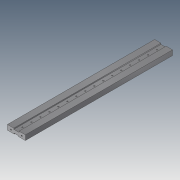
# Autodesk Inventor part: Zcolumn
Saved by Autodesk Inventor 2019 (Build 230136000, 136)
## iProperties
Created: 2018-10-03
Part Number: Zcolumn
Material: Aluminum 6061-AHC
Document SubType Name: Modeling
Designer: LillaHunden
Density: 2.7 g/cm^3
Appearance: Aluminum - Dark
Mass: 595.165 g
Surface Area: 512.389 cm^2
Volume: 220.432 cm^3
Author: LillaHunden
Autodesk Inventor part; units mm, degrees
ref_plane "YZ Plane" through (0, 0, 0) normal (1, 0, 0) x (0, 1, 0)
ref_plane "XZ Plane" through (0, 0, 0) normal (0, 1, 0) x (-1, 0, 0)
ref_plane "XY Plane" through (0, 0, 0) normal (0, 0, 1) x (1, 0, 0)
sketch "Sketch1" plane through (0, 0, 0) normal (0, 0, 1) x (1, 0, 0)
  line L0 (-83.9793, 29.5203) -> (-133.9793, 29.5203)
  line L1 (-133.9793, 29.5203) -> (-133.9793, 43.2703)
  line L2 (-133.9793, 43.2703) -> (-83.9793, 43.2703)
  line L3 (-83.9793, 43.2703) -> (-83.9793, 29.5203)
  point P0 (0, 0)
  dimension "d0" = 50
  dimension "d1" = 13.75
  constraints: 8 end point, 2 parallel, 1 horizontal, 1 perpendicular
  measures "d0" distance of L1.end L2.end
  measures "d1" distance of L0.end L1.end
extrude "Extrusion1" add sketch "Sketch1" along normal blind 410
sketch "Sketch2" plane through (-133.9793, 43.2703, 0) normal (0, 1, 0) x (1, 0, 0)
  line L0 (50, 0) -> (0, 0) projected
  line L1 (32.3, -410) -> (17.7, -410)
  line L2 (17.7, -410) -> (17.7, 0)
  line L3 (17.7, 0) -> (32.3, 0)
  line L4 (32.3, 0) -> (32.3, -410)
  line L5 (50, -410) -> (0, -410) projected
  point P0 (133.9793, 0)
  point P1 (25, -410)
  dimension "d4" = 14.6
  constraints: 8 end point, 2 midpoint, 2 parallel, 1 horizontal, 1 perpendicular, 1 point on line
  measures "d4" distance between parallel lines of L4 L2
extrude "Extrusion2" cut sketch "Sketch2" against normal blind 3
sketch "Sketch3" plane through (-133.9793, 29.5203, 0) normal (0, -1, 0) x (1, 0, 0)
  line L0 (17.7, 410) -> (0, 410) projected
  line L1 (17.7, 0) -> (32.3, 0) projected
  line L2 (18.9, 410) -> (31.1, 410)
  line L3 (31.1, 410) -> (31.1, 0)
  line L4 (31.1, 0) -> (18.9, 0)
  line L5 (18.9, 0) -> (18.9, 410)
  line L6 (0, 410) -> (50, 410) projected
  point P0 (133.9793, 0)
  point P1 (25, 410)
  dimension "d7" = 12.2
  constraints: 8 end point, 2 midpoint, 2 parallel, 2 point on line, 1 horizontal, 1 perpendicular
  measures "d7" distance of L3.end L4.end
extrude "Extrusion3" cut sketch "Sketch3" against normal blind 2
sketch "Sketch5" plane through (0, 0, 410) normal (0, 0, 1) x (1, 0, 0)
  point P0 (-93.9793, 35.7703)
  point P1 (-123.9793, 35.7703)
hole "Hole2" at (-93.9793, 35.7703, 410) at (-123.9793, 35.7703, 410) direction (0, 0, -1) diameter 3.242 depth 7.6214 tip angle 120 thread size "M4x0.7" class "6H" standard "ISO Metric profile"
ref_plane "Work Plane1" through (-108.9793, 29.5203, 0) normal (-1, 0, 0) x (0, 0, 1)
sketch "Sketch7" plane through (-133.9793, 31.5203, 0) normal (0, -1, 0) x (1, 0, 0)
  point P0 (25, 319)
  point P1 (25, 294)
  point P2 (25, 269)
  point P3 (25, 244)
  point P4 (25, 219)
  point P5 (25, 194)
  point P6 (25, 169)
  point P7 (25, 144)
  point P8 (25, 119)
  point P9 (25, 94)
  point P10 (25, 69)
  point P11 (25, 44)
  point P12 (25, 19)
  point P13 (25, 344)
  point P14 (25, 369)
  point P15 (25, 394)
sketch "Sketch8" plane through (-133.9793, 31.5203, 0) normal (0, -1, 0) x (1, 0, 0)
  point P0 (25, 393)
  point P1 (25, 368)
  point P2 (25, 343)
  point P3 (25, 318)
  point P4 (25, 293)
  point P5 (25, 268)
  point P6 (25, 243)
  point P7 (25, 218)
  point P8 (25, 193)
  point P9 (25, 168)
  point P10 (25, 143)
  point P11 (25, 118)
  point P12 (25, 93)
  point P13 (25, 68)
  point P14 (25, 43)
  point P15 (25, 18)
hole "Hole5" at (-108.9793, 31.5203, 393) at (-108.9793, 31.5203, 368) at (-108.9793, 31.5203, 343) at (-108.9793, 31.5203, 318) at (-108.9793, 31.5203, 293) at (-108.9793, 31.5203, 268) at (-108.9793, 31.5203, 243) at (-108.9793, 31.5203, 218) at (-108.9793, 31.5203, 193) at (-108.9793, 31.5203, 168) at (-108.9793, 31.5203, 143) at (-108.9793, 31.5203, 118) at (-108.9793, 31.5203, 93) at (-108.9793, 31.5203, 68) at (-108.9793, 31.5203, 43) at (-108.9793, 31.5203, 18) direction (0, 1, 0) diameter 3.4 depth 8.75
ref_plane "Work Plane2" through (-83.9793, 29.5203, 0) normal (0, -1, 0) x (1, 0, 0)
sketch "Sketch9" plane through (0, 0, 0) normal (0, 0, -1) x (-1, 0, 0)
  line L0 (83.9793, 43.2703) -> (83.9793, 29.5203) projected
  line L1 (83.9793, 36.3953) -> (133.9793, 36.3953) construction
  line L2 (133.9793, 29.5203) -> (133.9793, 43.2703) projected
  line L3 (101.6793, 43.2703) -> (83.9793, 43.2703) construction
  line L4 (133.9793, 43.2703) -> (116.2793, 43.2703) construction
  point P0 (0, 0)
  point P1 (92.8293, 36.3953)
  point P2 (125.1293, 36.3953)
  point P3 (108.9793, 36.3953)
  point P4 (92.8293, 43.2703)
  point P5 (125.1293, 43.2703)
  constraints: 5 midpoint, 2 end point, 2 point on line, 2 vertical alignment
hole "Hole7" at (-92.8293, 36.3953, 0) at (-108.9793, 36.3953, 0) at (-125.1293, 36.3953, 0) direction (0, 0, 1) diameter 4.134 depth 14.2 thread size "M5x0.8" class "6H" standard "ISO Metric profile"
body "Solid1"
